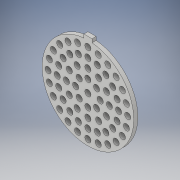
# Autodesk Inventor part: Матрица
Saved by Autodesk Inventor 2019 (Build 230136000, 136)
## iProperties
Created: 2019-04-26
Part Number: Матрица
Material: Типовые
Document SubType Name: Modeling
Designer: BarmanKaktus
Density: 1 g/cm^3
Appearance: По умолчанию
Author: BarmanKaktus
Autodesk Inventor part; units mm, degrees
ref_plane "YZ Plane" through (0, 0, 0) normal (1, 0, 0) x (0, 1, 0)
ref_plane "XZ Plane" through (0, 0, 0) normal (0, 1, 0) x (-1, 0, 0)
ref_plane "XY Plane" through (0, 0, 0) normal (0, 0, 1) x (1, 0, 0)
sketch "Эскиз1" plane through (0, 0, 0) normal (0, 0, 1) x (1, 0, 0)
  circle A0 centre (0, 0) radius 22.4
  line L0 (-2, 24) -> (2, 24)
  line L1 (2, 24) -> (2, 21)
  line L2 (2, 21) -> (-2, 21)
  line L3 (-2, 21) -> (-2, 24)
  dimension "d0" = 44.8
  dimension "d2" = 4
  dimension "d3" = 3
  dimension "d4" = 2
  dimension "d5" = 21
  constraints: 8 end point, 2 parallel, 1 centre point, 1 coincident, 1 horizontal, 1 perpendicular
  measures "d0" diameter of A0
  measures "d2" distance of L1.end L2.end
  measures "d3" distance of L0.end L1.end
  measures "d4" distance from line of point (0, 0) L1
  measures "d5" distance from line of point (0, 0) L2
extrude "Выдавливание1" add sketch "Эскиз1" along normal blind 2
sketch "Эскиз2" plane through (0, 0, 2) normal (0, 0, 1) x (1, 0, 0)
  circle A0 centre (0, 0) radius 22.4
  circle A1 centre (0, 0) radius 1.5
  circle A2 centre (0, -6) radius 1.5
  circle A3 centre (4.2426, -4.2426) radius 1.5
  circle A4 centre (6, 0) radius 1.5
  circle A5 centre (4.2426, 4.2426) radius 1.5
  circle A6 centre (0, 6) radius 1.5
  circle A7 centre (-4.2426, 4.2426) radius 1.5
  circle A8 centre (-6, 0) radius 1.5
  circle A9 centre (-4.2426, -4.2426) radius 1.5
  dimension "d8" = 3
  dimension "d9" = 3
  dimension "d10" = 6
  dimension "d13" = 360
  constraints: 10 centre point, 2 coincident, 17 other
  measures "d8" diameter of A1
  measures "d9" diameter of A2
  measures "d10" distance of point (0, 0) A2.centre
extrude "Выдавливание2" cut sketch "Эскиз2" against normal blind 2 contours A1 | A2 | A3 | A4 | A5 | A6 | A7 | A8 | A9
sketch "Эскиз3" plane through (0, 0, 2) normal (0, 0, 1) x (1, 0, 0)
  circle A0 centre (0, -10.5) radius 1.5
  circle A1 centre (5.25, -9.0933) radius 1.5
  circle A2 centre (9.0933, -5.25) radius 1.5
  circle A3 centre (10.5, 0) radius 1.5
  circle A4 centre (9.0933, 5.25) radius 1.5
  circle A5 centre (5.25, 9.0933) radius 1.5
  circle A6 centre (0, 10.5) radius 1.5
  circle A7 centre (-5.25, 9.0933) radius 1.5
  circle A8 centre (-9.0933, 5.25) radius 1.5
  circle A9 centre (-10.5, 0) radius 1.5
  circle A10 centre (-9.0933, -5.25) radius 1.5
  circle A11 centre (-5.25, -9.0933) radius 1.5
  point P0 (0, 0)
  dimension "d17" = 3
  dimension "d18" = 10.5
  dimension "d21" = 360
  constraints: 12 centre point, 25 other
  measures "d17" diameter of A0
  measures "d18" distance of point (0, 0) A0.centre
extrude "Выдавливание3" cut sketch "Эскиз3" along normal blind 2
extrude "Выдавливание4" cut sketch "Эскиз3" against normal blind 2
sketch "Эскиз4" plane through (0, 0, 2) normal (0, 0, 1) x (1, 0, 0)
  circle A0 centre (0, -15) radius 1.5
  point P0 (0, 0)
  dimension "d27" = 3
  dimension "d28" = 15
  constraints: 1 centre point
  measures "d27" diameter of A0
  measures "d28" distance of point (0, 0) A0.centre
extrude "Выдавливание5" cut sketch "Эскиз4" against normal blind 2
pattern_circular "Круговой массив1" count 20 over 360 about axis through (0, 0, 2) along (0, 0, -1) of "Выдавливание5"
sketch "Эскиз5" plane through (0, 0, 2) normal (0, 0, 1) x (1, 0, 0)
  circle A0 centre (0, -19.5) radius 1.5
  point P0 (0, 0)
  dimension "d34" = 3
  dimension "d35" = 19.5
  constraints: 1 centre point
  measures "d34" diameter of A0
  measures "d35" distance of point (0, 0) A0.centre
extrude "Выдавливание6" cut sketch "Эскиз5" against normal blind 2
pattern_circular "Круговой массив2" count 24 over 360 about axis through (0, 0, 2) along (0, 0, -1) of "Выдавливание6"
